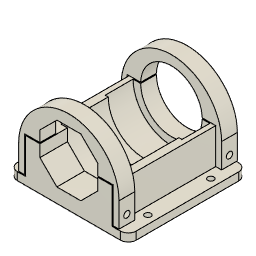
Ball+Valve+Mount+(Marine) (Autodesk Fusion 360 design; units mm, degrees)
Autodesk Fusion 360 part; units mm, degrees
sketch "Sketch2" plane through (0, 0, 0) normal (0, 1, 0) x (1, 0, 0)
  line L0 (0, -20) -> (0, -2.5) construction
  line L1 (2.5, 0) -> (20, 0) construction
  line L2 (15.625, 0) -> (15.625, -8)
  line L3 (15.625, -8) -> (19.5, -8)
  line L4 (19.5, -8) -> (19.5, -22.15)
  line L5 (19.5, -22.15) -> (17.95, -22.15)
  line L6 (17.95, -22.15) -> (17.95, -46.15)
  line L7 (17.95, -46.15) -> (14.7, -46.15)
  line L8 (14.7, -46.15) -> (14.7, -60.15)
  line L9 (14.7, -60.15) -> (22, -60.15)
  line L10 (22, -60.15) -> (22, 0)
  line L11 (22, 0) -> (15.625, 0)
  dimension "d1" = 15.625
  dimension "d2" = 8
  dimension "d3" = 19.5
  dimension "d4" = 14.15
  dimension "d5" = 17.95
  dimension "d6" = 24
  dimension "d7" = 14
  dimension "d8" = 14.7
  dimension "d9" = 2.5
  constraint perpendicular L1 L2
  constraint perpendicular L2 L3
  constraint perpendicular L1 L4
  constraint coincident L1 L2.start
  constraint perpendicular L4 L5
  constraint perpendicular L5 L6
  constraint perpendicular L6 L7
  constraint perpendicular L7 L8
  constraint perpendicular L8 L9
  constraint perpendicular L9 L10
  constraint perpendicular L2 L11
  measures "d1" distance of L0 L2
  measures "d2" distance of L2.start L2.end
  measures "d3" distance of L0 L4
  measures "d4" distance of L3.end L4.end
  measures "d5" distance of L0 L6
  measures "d6" distance of L5.end L6.end
  measures "d7" distance of L7.end L8.end
  measures "d8" distance of L0 L8
  measures "d9" distance of L4 L10
revolve "Revolve1" add sketch "Sketch2" angle 180 about axis through (0, 0, 20) along (0, 0, -1) makes body 1
sketch "Sketch3" plane through (0, 0, 60.15) normal (0, 0, 1) x (1, 0, 0)
  line L0 (22, 0) -> (14.7, 0)
  arc A0 (-14.7, 0) -> (14.7, 0) centre (0, 0) ccw
  line L1 (-14.7, 0) -> (-22, 0)
  arc A1 (-22, 0) -> (22, 0) centre (0, 0) ccw
  line L2 (-30.2, -22) -> (30.2, -22)
  line L3 (14.7, 6.0889) -> (6.0889, 14.7)
  line L4 (6.0889, 14.7) -> (-6.0889, 14.7)
  line L5 (-6.0889, 14.7) -> (-14.7, 6.0889)
  line L6 (-14.7, 6.0889) -> (-14.7, -6.0889)
  line L7 (-14.7, -6.0889) -> (-6.0889, -14.7)
  line L8 (-6.0889, -14.7) -> (6.0889, -14.7)
  line L9 (6.0889, -14.7) -> (14.7, -6.0889)
  line L10 (14.7, -6.0889) -> (14.7, 6.0889)
  line L11 (-30.2, -22) -> (-30.2, -18)
  line L12 (-30.2, -18) -> (-22, -18)
  line L13 (30.2, -22) -> (30.2, -18)
  line L14 (30.2, -18) -> (22, -18)
  line L15 (-22, 0) -> (-22, -18)
  line L16 (22, 0) -> (22, -18)
  line L17 (-25.5, -17.5) -> (-22.5, -17.5)
  line L18 (-22.5, -17.5) -> (-22.5, 0.5)
  line L19 (-22.5, 0.5) -> (-14.7, 0.5)
  line L20 (-25.5, -17.5) -> (-25.5, -5)
  line L21 (0, 2.5) -> (0, 20) construction
  arc A2 (25.5, -5) -> (-25.5, -5) centre (0, -5) ccw
  line L22 (22.5, 0.5) -> (14.7, 0.5)
  line L23 (22.5, -17.5) -> (22.5, 0.5)
  line L24 (25.5, -17.5) -> (22.5, -17.5)
  line L25 (25.5, -17.5) -> (25.5, -5)
  dimension "d12" = 4
  dimension "d13" = 8.2
  dimension "d14" = 0.5
  dimension "d15" = 0.5
  dimension "d16" = 0.5
  dimension "d17" = 3
  dimension "d18" = 5
  dimension "d19" = 25.5
  constraint horizontal L2
  constraint tangent A1 L2
  constraint coincident A0.centre A1.centre
  constraint perpendicular L0 L10
  constraint coincident L0.end L10
  constraint perpendicular L2 L11
  constraint perpendicular L11 L12
  constraint perpendicular L2 L13
  constraint perpendicular L13 L14
  constraint equal L12 L14
  constraint equal L11 L13
  constraint coincident L1.end A1.start
  constraint coincident L12 L15.end
  constraint tangent A1 L15
  constraint coincident L0.start A1.end
  constraint coincident L14 L16.end
  constraint tangent A1 L16
  constraint coincident L12.end L15.end
  constraint coincident L14.end L16.end
  constraint horizontal L17
  constraint perpendicular L17 L18
  constraint coincident L6 L19.end
  constraint perpendicular L6 L19
  constraint perpendicular L17 L20
  constraint symmetric L17.start L21 L24.start
  constraint symmetric L17.end L21 L23.start
  constraint symmetric L18.end L21 L22.start
  constraint symmetric L19.end L21 L22.end
  constraint symmetric L20.end L21 A2.start
  constraint coincident A2.start L25.end
  measures "d12" distance of L2.start L11.end
  measures "d13" distance of L11.end L12.end
  measures "d14" distance of L12 L17
  measures "d15" distance of L15 L18
  measures "d16" distance of L1 L19
  measures "d17" distance of L17.start L17.end
  measures "d18" distance of A0.centre A2.centre
  measures "d19" radius of A2
extrude "Extrude1" add sketch "Sketch3" against normal up to surface (60.15 mm away) contours A1 L2 L13 L14 L16 | A1 L2 L11 L12 L15 bodies 1
extrude "Extrude2" cut sketch "Sketch3" against normal up to surface (14 mm away) contours A0 L9 L10 | A0 L8 L9 | A0 L7 L8 | A0 L6 L7 bodies 1
sketch "Sketch4" plane through (0, 0, 0) normal (0, 0, -1) x (-1, 0, 0)
  line L0 (-15.625, 0) -> (-22, 0)
  line L1 (-22, 0) -> (-22, -18)
  line L2 (-22, -18) -> (-30.2, -18)
  line L3 (-30.2, -18) -> (-30.2, -22)
  line L4 (-30.2, -22) -> (30.2, -22)
  line L5 (30.2, -22) -> (30.2, -18)
  line L6 (30.2, -18) -> (22, -18)
  line L7 (22, -18) -> (22, 0)
  line L8 (22, 0) -> (15.625, 0)
  arc A0 (-15.625, 0) -> (15.625, 0) centre (0, 0) ccw
  arc A1 (25.5, -5) -> (-25.5, -5) centre (0, -5) ccw
  line L9 (-25.5, -17.5) -> (-25.5, -5)
  line L10 (-25.5, -17.5) -> (-22.5, -17.5)
  line L11 (-22.5, -17.5) -> (-22.5, 0.5)
  line L12 (-22.5, 0.5) -> (-14.7, 0.5)
  line L13 (22.5, 0.5) -> (14.7, 0.5)
  line L14 (22.5, -17.5) -> (22.5, 0.5)
  line L15 (25.5, -17.5) -> (25.5, -5)
  line L16 (25.5, -17.5) -> (22.5, -17.5)
  arc A2 (-15.625, 0) -> (15.625, 0) centre (0, 0) ccw
  circle A3 centre (0, 0) radius 15.625
  constraint concentric A0 A3
  constraint coincident L8.end A3
extrude "Extrude3" add sketch "Sketch4" against normal up to surface (8 mm away) separate body contours A1 L9 L10 L11 L12 L13 L14 L15 L16 A3 makes body 2
extrude "Extrude4" add sketch "Sketch3" against normal blind 8 separate body contours L3 L4 L5 L6 L10 L17 L18 L19 L20 A2 L22 L23 L24 L25 makes body 3
sketch "Sketch6" plane through (-22, 0, 0) normal (-1, 0, 0) x (0, 0, 1)
  line L0 (0, 0) -> (0, -18)
  line L1 (0, -18) -> (60.15, -18)
  line L2 (60.15, -18) -> (60.15, 0)
  line L3 (60.15, 0) -> (0, 0)
  line L4 (8, -17.5) -> (8, -5)
  line L5 (8, -5) -> (0, -5)
  line L6 (0, -5) -> (0, -17.5)
  line L7 (0, -17.5) -> (8, -17.5)
  line L8 (60.15, -17.5) -> (60.15, -5)
  line L9 (60.15, -5) -> (52.15, -5)
  line L10 (52.15, -5) -> (52.15, -17.5)
  line L11 (52.15, -17.5) -> (60.15, -17.5)
  line L12 (30.075, 0) -> (30.075, -18) construction
  line L13 (4, -5) -> (4, -17.5) construction
  line L14 (56.15, -5) -> (56.15, -17.5) construction
  circle A0 centre (4, -13) radius 1.6
  circle A1 centre (4, -12.5) radius 2.5
  circle A2 centre (56.15, -13) radius 1.6
  circle A3 centre (56.15, -12.5) radius 2.5
  dimension "d30" = 3.2
  dimension "d31" = 5
  dimension "d34" = 5
  dimension "d35" = 3.2
  dimension "d53" = 5
  dimension "d54" = 4.5
  dimension "d55" = 5
  dimension "d56" = 4.5
  constraint midpoint L3 L12.start
  constraint midpoint L1 L12.end
  constraint midpoint L5 L13.start
  constraint midpoint L7 L13.end
  constraint midpoint L9 L14.start
  constraint midpoint L11 L14.end
  constraint coincident L14 A2.centre
  constraint coincident L13 A0.centre
  constraint coincident L14 A3.centre
  measures "d30" diameter of A0
  measures "d31" diameter of A1
  measures "d34" diameter of A3
  measures "d35" diameter of A2
  measures "d53" distance of L7 A1.centre
  measures "d54" distance of L7 A0.centre
  measures "d55" distance of L11 A3.centre
  measures "d56" distance of L11 A2.centre
sketch "Sketch7" plane through (22, 0, 0) normal (1, 0, 0) x (0, 0, -1)
  line L0 (0, -18) -> (0, 0)
  line L1 (0, 0) -> (-60.15, 0)
  line L2 (-60.15, 0) -> (-60.15, -18)
  line L3 (-60.15, -18) -> (0, -18)
  circle A0 centre (-4, -12.5) radius 2.5
  circle A1 centre (-4, -13) radius 1.6
  circle A2 centre (-56.15, -13) radius 1.6
  circle A3 centre (-56.15, -12.5) radius 2.5
extrude "Extrude5" cut sketch "Sketch6" along normal up to surface (3.5 mm away) contours A0 | A2 bodies 2 3
extrude "Extrude6" cut sketch "Sketch7" along normal up to surface (3.5 mm away) contours A1 | A2 bodies 2 3
extrude "Extrude7" cut sketch "Sketch6" against normal blind 5 contours A0 | A1 | A2 | A3 bodies 1
extrude "Extrude8" cut sketch "Sketch7" against normal blind 5 contours A0 | A1 | A2 | A3 bodies 1
sketch "Sketch8" plane through (0, -18, 0) normal (0, 1, 0) x (-1, 0, 0)
  line L0 (22, 0) -> (30.2, 0)
  line L1 (30.2, 0) -> (30.2, 60.15)
  line L2 (30.2, 60.15) -> (22, 60.15)
  line L3 (22, 60.15) -> (22, 0)
  line L4 (30.2, 30.075) -> (22, 30.075) construction
  circle A0 centre (26.1, 14.075) radius 1.55
  line L5 (0, 20) -> (0, 2.5) construction
  circle A1 centre (-26.1, 14.075) radius 1.55
  circle A2 centre (-26.1, 46.075) radius 1.55
  circle A3 centre (26.1, 46.075) radius 1.55
  dimension "d44" = 16
  dimension "d47" = 26.1
  dimension "d48" = 3.1
  constraint midpoint L1 L4.start
  constraint midpoint L3 L4.end
  constraint symmetric A0 L5 A1
  constraint symmetric L4 A0 A3
  constraint symmetric L4 A1 A2
  measures "d44" distance of L4 A0.centre
  measures "d47" distance of A0.centre L5
  measures "d48" diameter of A0
extrude "Extrude9" cut sketch "Sketch8" against normal up to surface (4 mm away) contours A0 | A1 | A2 | A3 bodies 1
fillet "Fillet1" radius 4 4 edges at (30.2, -20, 0) (30.2, -20, 60.15) (-30.2, -20, 60.15) (-30.2, -20, 0) on bodies 1
equation "d34 = d31"
equation "d35 = d30"
equation "d55 = d53"
equation "d56 = d54"
named bodies: "BV Base", "Circle Strap", "Hex Strap"
